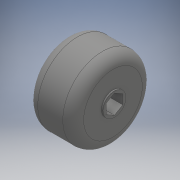
# Autodesk Inventor part: 38omuni14184
Saved by Autodesk Inventor 2018.2 (Build 222227000, 227)
## iProperties
Created: 2018-09-03
Part Number: 38omuni14184
Material: 一般
Document SubType Name: Modeling
Designer: シュンダイ
Density: 1 g/cm^3
Appearance: 滑らか - 黒
Author: シュンダイ
Autodesk Inventor part; units mm, degrees
ref_plane "YZ Plane" through (0, 0, 0) normal (1, 0, 0) x (0, 1, 0)
ref_plane "XZ Plane" through (0, 0, 0) normal (0, 1, 0) x (-1, 0, 0)
ref_plane "XY Plane" through (0, 0, 0) normal (0, 0, 1) x (1, 0, 0)
sketch "スケッチ1" plane through (0, 0, 0) normal (1, 0, 0) x (0, 1, 0)
  circle A0 centre (0, 0) radius 19.05
  dimension "d0" = 38.1
  constraints: 1 centre point, 1 coincident
  measures "d0" diameter of A0
extrude "押し出し1" add sketch "スケッチ1" along normal blind 22
hole "穴1" at (22, 0, 0) direction (-1, 0, 0) diameter 5.2 end through all
sketch "スケッチ2" plane through (22, 0, 0) normal (1, 0, 0) x (0, 0, -1)
  circle A0 centre (0, 0) radius 5.5
  dimension "d12" = 11
  constraints: 1 centre point, 1 coincident
  measures "d12" diameter of A0
extrude "押し出し2" add sketch "スケッチ2" along normal blind 0.7
sketch "スケッチ3" plane through (0, 0, 0) normal (-1, 0, 0) x (0, 0, 1)
  circle A0 centre (0, 0) radius 5.5
  dimension "d15" = 11
  constraints: 1 centre point, 1 coincident
  measures "d15" diameter of A0
extrude "押し出し3" add sketch "スケッチ3" along normal blind 0.7
fillet "フィレット1" radius 5 1 edges at (0, -19.05, 0)
fillet "フィレット2" radius 5 1 edges at (22, -19.05, 0)
sketch "スケッチ4" plane through (-0.7, 0, 0) normal (-1, 0, 0) x (0, 0, 1)
  line L0 (-2.3094, -4) -> (-4.6188, 0)
  line L1 (-4.6188, 0) -> (-2.3094, 4)
  line L2 (-2.3094, 4) -> (2.3094, 4)
  line L3 (2.3094, 4) -> (4.6188, 0)
  line L4 (4.6188, 0) -> (2.3094, -4)
  line L5 (2.3094, -4) -> (-2.3094, -4)
  point P0 (0, 0)
  point P1 (0, 0)
  point P2 (0, -4)
  constraints: 12 end point, 1 midpoint, 13 other
sketch "スケッチ5" plane through (22.7, 0, 0) normal (1, 0, 0) x (0, 0, -1)
  line L0 (2.3094, 4) -> (4.6188, 0)
  line L1 (4.6188, 0) -> (2.3094, -4)
  line L2 (2.3094, -4) -> (-2.3094, -4)
  line L3 (-2.3094, -4) -> (-4.6188, 0)
  line L4 (-4.6188, 0) -> (-2.3094, 4)
  line L5 (-2.3094, 4) -> (2.3094, 4)
  point P0 (0, 0)
  point P1 (0, 0)
  point P2 (0, 4)
  constraints: 12 end point, 1 midpoint, 13 other
extrude "押し出し4" cut sketch "スケッチ4" against normal blind 10
extrude "押し出し5" cut sketch "スケッチ5" against normal blind 10
